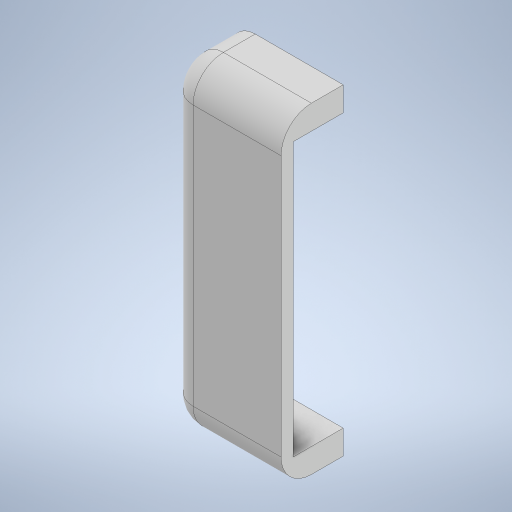
# Autodesk Inventor part: uchwyt_serw
Saved by Autodesk Inventor 2023 (Build 270158000, 158)
## iProperties
Created: 2023-08-17
Part Number: uchwyt_serw
Material: Ogólny
Document SubType Name: Modeling
Designer: Kamil
Density: 1 g/cm^3
Appearance: Domyślna
Author: Kamil
Autodesk Inventor part; units mm, degrees
ref_plane "YZ Plane" through (0, 0, 0) normal (1, 0, 0) x (0, 1, 0)
ref_plane "XZ Plane" through (0, 0, 0) normal (0, 1, 0) x (-1, 0, 0)
sketch "Szkic1" plane through (0, 0, 0) normal (0, 0, 1) x (1, 0, 0)
  line L0 (13.65, -45) -> (17, -45) projected
  line L1 (0.5, -45) -> (12.85, -45) projected
  line L2 (17, -25) -> (13.65, -25) projected
  line L3 (12.85, -25) -> (0.5, -25) projected
  line L4 (13.65, -20) -> (17, -20) projected
  line L5 (0.5, -20) -> (12.85, -20) projected
  line L6 (12.85, 0) -> (0.5, 0) projected
  line L7 (17, 0) -> (13.65, 0) projected
  line L8 (0, -25.5) -> (0, -44.5) projected
  line L9 (0, -0.5) -> (0, -19.5) projected
  line L10 (17.5, -12.6805) -> (17.5, -0.5) projected
  line L11 (17.5, -44.5) -> (17.5, -32.3195) projected
  line L12 (0, -45) -> (17.5, -45)
  line L13 (17.5, -45) -> (17.5, -49)
  line L14 (17.5, -49) -> (0, -49)
  line L15 (0, -49) -> (0, -45)
  line L16 (0, -20) -> (17.5, -20)
  line L17 (17.5, -20) -> (17.5, -25)
  line L18 (17.5, -25) -> (0, -25)
  line L19 (0, -25) -> (0, -20)
  line L20 (0, 0) -> (17.5, 0)
  line L21 (17.5, 0) -> (17.5, 4)
  line L22 (17.5, 4) -> (0, 4)
  line L23 (0, 4) -> (0, 0)
  line L24 (0, 4) -> (17.5, 4)
  line L25 (17.5, 4) -> (17.5, -49)
  line L26 (17.5, -49) -> (0, -49)
  line L27 (0, -49) -> (0, 4)
  dimension "d0" = 4
  dimension "d1" = 4
  constraints: 32 end point, 8 parallel, 4 horizontal, 4 perpendicular, 4 point on line
  measures "d0" distance of L12.end L13.end
  measures "d1" distance of L21.end L20.end
ref_plane "Płaszczyzna konstrukcyjna1" through (-42.5, -72.5, -8.25) normal (0, 0, 1) x (1, 0, 0)
extrude "Wyciągnięcie proste1" add sketch "Szkic1" against normal up to surface (8.25 mm away) contours L0 L12 L13 L14 L15 L1 | L18 L2 L3 L19 L16 L5 L4 L17 | L20 L7 L6 L23 L22 L21
sketch "Szkic2" plane through (0, 0, 0) normal (0, 0, 1) x (1, 0, 0)
  line L0 (0, 0) -> (17.5, 0) projected
  line L1 (17.5, 0) -> (17.5, 4) projected
  line L2 (17.5, 4) -> (0, 4) projected
  line L3 (0, 4) -> (0, 0) projected
  line L4 (0, -25) -> (17.5, -25) projected
  line L5 (17.5, -25) -> (17.5, -20) projected
  line L6 (17.5, -20) -> (0, -20) projected
  line L7 (0, -20) -> (0, -25) projected
  line L8 (0, -49) -> (17.5, -49) projected
  line L9 (17.5, -49) -> (17.5, -45) projected
  line L10 (17.5, -45) -> (0, -45) projected
  line L11 (0, -45) -> (0, -49) projected
  line L12 (0, 4) -> (17.5, 4) projected
  line L13 (17.5, 4) -> (0, 4)
  line L14 (0, 4) -> (0, -49)
  line L15 (0, -49) -> (17.5, -49)
  line L16 (17.5, -49) -> (17.5, 4)
  constraints: 8 end point, 2 parallel, 1 horizontal, 1 perpendicular
extrude "Wyciągnięcie proste2" add sketch "Szkic2" along normal blind 2
sketch "Szkic3" plane through (0, 0, 2) normal (0, 0, 1) x (1, 0, 0)
  line L0 (17.5, -45) -> (0, -45) projected
  line L1 (0, 4) -> (0, -49) projected
  line L2 (0, -49) -> (17.5, -49) projected
  line L3 (17.5, -49) -> (17.5, 4) projected
  line L4 (0, -25) -> (17.5, -25) projected
  line L5 (17.5, -20) -> (0, -20) projected
  line L6 (0, 0) -> (17.5, 0) projected
  line L7 (17.5, 4) -> (0, 4) projected
  point P0 (13.5, -47)
  point P1 (4, -47)
  point P2 (13.5, -22.5)
  point P3 (4, -22.5)
  point P4 (13.5, 2)
  point P5 (4, 2)
  dimension "d6" = 2
  dimension "d7" = 2
  dimension "d8" = 2.5
  dimension "d9" = 2.5
  dimension "d10" = 2
  dimension "d11" = 2
  dimension "d12" = 4
  dimension "d13" = 4
  dimension "d14" = 4
  dimension "d15" = 4
  dimension "d16" = 4
  dimension "d17" = 4
  measures "d6" distance from line of point (13.5, 2) L7
  measures "d7" distance from line of point (4, 2) L7
  measures "d8" distance from line of point (13.5, -22.5) L5
  measures "d9" distance from line of L5 point (4, -22.5)
  measures "d10" distance from line of point (13.5, -47) L2
  measures "d11" distance from line of point (4, -47) L2
  measures "d12" distance from line of point (13.5, -47) L3
  measures "d13" distance from line of L1 point (4, -47)
  measures "d14" distance from line of L3 point (13.5, -22.5)
  measures "d15" distance from line of L3 point (13.5, 2)
  measures "d16" distance from line of point (4, -22.5) L1
  measures "d17" distance from line of point (4, 2) L1
hole "Otwór1" at (13.5, -47, 2) at (4, -47, 2) at (13.5, -22.5, 2) at (4, -22.5, 2) at (13.5, 2, 2) at (4, 2, 2) direction (0, 0, -1) diameter 2 end through all
sketch "Szkic4" plane through (0, 0, 2) normal (0, 0, 1) x (1, 0, 0)
  circle A0 centre (13.5, 2) radius 1 projected
  circle A1 centre (13.5, -22.5) radius 1 projected
  circle A2 centre (13.5, -47) radius 1 projected
  circle A3 centre (4, -47) radius 1 projected
  circle A4 centre (4, -22.5) radius 1 projected
  circle A5 centre (4, 2) radius 1 projected
  line L0 (17.5, -49) -> (17.5, 4) projected
  line L1 (17.5, 4) -> (0, 4) projected
  line L2 (0, 4) -> (0, -49) projected
  line L3 (0, -49) -> (17.5, -49) projected
  point P0 (0, 0)
extrude "Wyciągnięcie proste3" add sketch "Szkic4" against normal blind 3 contours A0 | A1 | A2 | A3 | A4 | A5
fillet "Zaokrąglenie1" radius 5 2 edges at (8.75, 4, 2) (8.75, -49, 2)
sketch "Szkic5" plane through (0, -25, -8.25) normal (-1, 0, 0) x (0, 0, 1)
  arc A0 (5.25, -24) -> (10.25, -19) centre (5.25, -19) ccw projected
  line L0 (10.25, 24) -> (10.25, -19) projected
  arc A1 (10.25, 24) -> (5.25, 29) centre (5.25, 24) ccw projected
  line L1 (0, 29) -> (5.25, 29) projected
  line L2 (0, 25) -> (0, 29) projected
  line L3 (8.25, 25) -> (0, 25) projected
  line L4 (8.25, 25) -> (8.25, 5) projected
  line L5 (8.25, 5) -> (0, 5) projected
  line L6 (0, 0) -> (0, 5) projected
  line L7 (8.25, 0) -> (0, 0) projected
  line L8 (8.25, 0) -> (8.25, -20) projected
  line L9 (8.25, -20) -> (0, -20) projected
  line L10 (0, -24) -> (0, -20) projected
  line L11 (5.25, -24) -> (0, -24) projected
  line L12 (0, 25) -> (0, -20)
  constraints: 3 end point
extrude "Wyciągnięcie proste4" add sketch "Szkic5" along normal blind 1
fillet "Zaokrąglenie2" radius 4 5 edges at (-1, 4, -5.625) (-1, -22.5, 2) (-1, -47.5355, 0.5355) (-1, -49, -5.625) (-1, 2.5355, 0.5355)
sketch "Szkic6" plane through (17.5, -25, -8.25) normal (0, 0, -1) x (-1, 0, 0)
  circle A0 centre (13.5, -22) radius 1 projected
  circle A1 centre (4, -22) radius 1 projected
  circle A2 centre (13.5, 27) radius 1 projected
  circle A3 centre (4, 27) radius 1 projected
  circle A4 centre (4, 2.5) radius 1 projected
  circle A5 centre (13.5, 2.5) radius 1 projected
  arc A6 (18.5, 25) -> (14.5, 29) centre (14.5, 25) ccw projected
  line L0 (14.5, 29) -> (0, 29) projected
  line L1 (0, 29) -> (0, 25) projected
  line L2 (0, 25) -> (17.5, 25) projected
  line L3 (17.5, 25) -> (17.5, 5) projected
  line L4 (17.5, 5) -> (0, 5) projected
  line L5 (0, 5) -> (0, 0) projected
  line L6 (0, 0) -> (17.5, 0) projected
  line L7 (17.5, 0) -> (17.5, -20) projected
  line L8 (17.5, -20) -> (0, -20) projected
  line L9 (0, -20) -> (0, -24) projected
  line L10 (0, -24) -> (14.5, -24) projected
  arc A7 (14.5, -24) -> (18.5, -20) centre (14.5, -20) ccw projected
  line L11 (18.5, 25) -> (18.5, -20) projected
  line L12 (17.5, 0) -> (0, 0) projected
  line L13 (0, 5) -> (17.5, 5)
  line L14 (17.5, 5) -> (17.5, 0)
  line L15 (17.5, 0) -> (0, 0)
  line L16 (0, 0) -> (0, 5)
  constraints: 8 end point, 2 parallel, 1 horizontal, 1 perpendicular
extrude "Wyciągnięcie proste5" cut sketch "Szkic6" against normal up to surface (8.25 mm away) contours A4 | A5 | L14 L6 L5 L4
